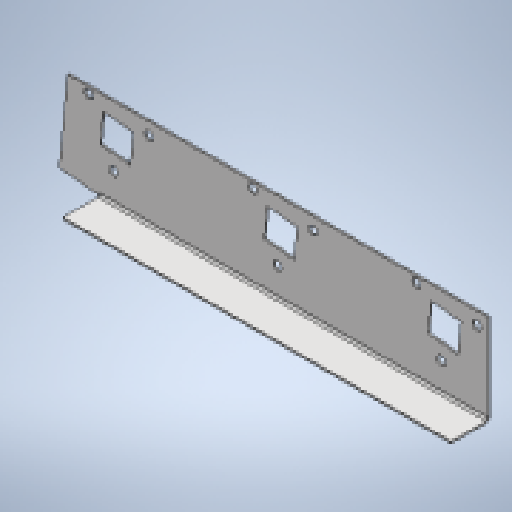
# Autodesk Inventor part: MNT-CDF-501 box
Saved by Autodesk Inventor 2025.1 (Build 291241020, 241B)
## iProperties
Created: 2025-01-13
Part Number: MNT-CDF-501 box
Material: Stainless Steel
Description: DIE16(5)|\ 90°|corrY -___°|X_____|bom___
Document SubType Name: Sheet Metal
Designer: user
Stock Number: МОО 305 шпангоут борт
Mass: 1762.25 g
Surface Area: 2283.33 cm^2
Volume: 220.281 cm^3
Density: 8 g/cm^3
Sheet Metal Rule: AISI304 2mm Die16
Sheet Metal Width: 146.202 mm
Sheet Metal Length: 606.604 mm
Sheet Metal Area: 88686.698 mm^2
Appearance: Default
Flat Pattern Width: 14.6202 cm
Flat Pattern Length: 60.6604 cm
Flat Pattern Area: 886.867 cm^2
Author: user
Autodesk Inventor part; units mm, degrees
ref_plane "YZ Plane" through (0, 0, 0) normal (1, 0, 0) x (0, 1, 0)
ref_plane "XZ Plane" through (0, 0, 0) normal (0, 1, 0) x (-1, 0, 0)
ref_plane "XY Plane" through (0, 0, 0) normal (0, 0, 1) x (1, 0, 0)
sketch "Sketch1" plane through (0, 0, 0) normal (0, 0, 1) x (1, 0, 0)
  line L0 (0, -22.5) -> (560, -22.5)
  line L1 (560, -22.5) -> (560, 22.5)
  line L2 (560, 22.5) -> (0, 22.5)
  line L3 (0, 22.5) -> (0, -22.5)
  line L4 (0, -22.5) -> (560, 22.5) construction
  line L5 (560, -22.5) -> (0, 22.5) construction
  point P0 (0, 0)
  point P1 (0, 0)
  dimension "d154" = 560
  dimension "d155" = 45
  measures "d154" distance of L1.end L2.end
  measures "d155" distance of L0.end L1.end
extrude "Plate3" add sketch "Sketch1" along normal blind 2
sketch "Sketch7" plane through (0, 20.5, 0) normal (0, 1, 0) x (-1, 0, 0)
  line L0 (-560, 0) -> (0, 0)
  line L1 (0, 0) -> (0, 105)
  line L2 (0, 105) -> (-560, 105)
  line L3 (-560, 105) -> (-560, 0)
  constraints: 6 end point, 1 horizontal, 1 perpendicular, 1 vertical
edge flange "Flange3" height 105 angle 90 thickness 2 bend radius 2.75 thickness toward (0, 1, 0) relief round relief width 2 relief depth 1 edges at (280, 22.5, 2) wall of the first edge with corners at (560, 20.5, 0) (0, 20.5, 0) (0, 20.5, 105) (560, 20.5, 105)
bend "Bend3"
corner "Corner3"
sketch "Sketch11" plane through (0, 20.5, 105) normal (0, -1, 0) x (1, 0, 0)
  line L0 (0, -100.25) -> (560, -100.25) projected
  line L1 (560, -100.25) -> (560, 0) projected
  line L2 (560, 0) -> (0, 0) projected
  line L3 (0, -100.25) -> (0, 0) projected
  line L4 (0, 0) -> (-23.7581, 0)
  line L5 (-23.7581, 0) -> (-49.4388, -103)
  line L6 (-49.4388, -103) -> (-1, -103)
  line L7 (-1, -103) -> (-1, -100.25)
  line L8 (-1, -100.25) -> (0, -100.25)
  line L9 (560, -103) -> (0, -103) projected
  line L10 (-1, -103) -> (-46.6039, -91.6297)
  point P0 (0, -105)
  dimension "d193" = 1
  dimension "d194" = 23.7581
  dimension "d195" = 14
  dimension "d203" = 47
  constraints: 12 end point, 3 perpendicular, 1 collinear, 1 horizontal, 1 parallel, 1 point on line
  measures "d193" distance of L7.end L0.start
  measures "d194" distance of L2.end L4.end
  measures "d195" angle of L3 L5
  measures "d203" distance of L6.end L10.end
extrude "Extrusion6" add sketch "Sketch11" against normal up to surface (2 mm away) contours L8 L7 L10 L5 L4 L3
sketch "Sketch12" plane through (560, 20.5, 4.75) normal (0, -1, 0) x (1, 0, 0)
  line L0 (-511.4632, 69.8575) -> (-545.4236, 78.3248)
  line L1 (-545.4236, 78.3248) -> (-553.8908, 44.3644)
  line L2 (-553.8908, 44.3644) -> (-519.9305, 35.8972)
  line L3 (-519.9305, 35.8972) -> (-511.4632, 69.8575)
  line L4 (-511.4632, 69.8575) -> (-553.8908, 44.3644) construction
  line L5 (-545.4236, 78.3248) -> (-519.9305, 35.8972) construction
  circle A0 centre (-541.1443, 23.1506) radius 5.05
  circle A1 centre (-492.6686, 72.9011) radius 5.05
  circle A2 centre (-560.5893, 89.8356) radius 5.05
  line L6 (-492.6686, 72.9011) -> (-560.5893, 89.8356) construction
  line L7 (-560.5893, 89.8356) -> (-541.1443, 23.1506) construction
  line L8 (-541.1443, 23.1506) -> (-492.6686, 72.9011) construction
  line L9 (-528.4434, 74.0911) -> (-541.1443, 23.1506) construction
  line L10 (-583.7581, 100.25) -> (-606.6039, 8.6203) projected
  point P0 (-560, -4.75)
  point P1 (-532.677, 57.111)
  point P2 (-543.753, 12.6876)
  dimension "d206" = 35
  dimension "d207" = 35
  dimension "d208" = 10.1
  dimension "d209" = 70
  dimension "d210" = 60
  dimension "d211" = 25
  dimension "d213" = 12
  dimension "d214" = 60
  constraints: 20 end point, 4 parallel, 3 centre point, 3 midpoint, 1 equal radius, 1 perpendicular, 1 point on line, 2 other
  measures "d206" distance of L5.end L4.end
  measures "d207" distance of L4.end L5.start
  measures "d208" diameter of A0
  measures "d209" distance of L6.start L7.start
  measures "d210" distance from line of L9.end L6
  measures "d211" distance from line of L6 point (-532.677, 57.111)
  measures "d213" distance from line of L10.start L0
  measures "d214" distance from line of L10 point (-532.677, 57.111)
extrude "Cut1" cut sketch "Sketch12" against normal blind 2
pattern_linear "Rectangular Pattern5" count 4 spacing 160 along (1, 0, 0) of "Cut1"
body "Solid2"
